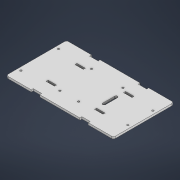
# Autodesk Inventor part: chassis
Saved by Autodesk Inventor 2021 (Build 250183000, 183)
## iProperties
Created: 2022-06-26
Part Number: chassis
Material: Generic
Document SubType Name: Modeling
Designer: phand
Density: 1 g/cm^3
Appearance: Default
Author: phand
Autodesk Inventor part; units mm, degrees
ref_plane "YZ Plane" through (0, 0, 0) normal (1, 0, 0) x (0, 1, 0)
ref_plane "XZ Plane" through (0, 0, 0) normal (0, 1, 0) x (-1, 0, 0)
ref_plane "XY Plane" through (0, 0, 0) normal (0, 0, 1) x (1, 0, 0)
sketch "Sketch1" plane through (0, 0, 0) normal (0, 1, 0) x (-1, 0, 0)
  line L0 (80, 45) -> (-80, 45)
  line L1 (-80, 45) -> (-80, -45)
  line L2 (-80, -45) -> (80, -45)
  line L3 (80, -45) -> (80, 45)
  line L4 (80, 45) -> (-80, -45) construction
  line L5 (-80, 45) -> (80, -45) construction
  point P0 (0, 0)
  dimension "d0" = 160
  dimension "d1" = 90
  constraints: 12 end point, 2 midpoint, 2 parallel, 1 horizontal, 1 perpendicular
  measures "d0" distance of L2.end L1.end
  measures "d1" distance of L1.end L0.end
extrude "Extrusion1" add sketch "Sketch1" along normal blind 3
sketch "Sketch2" plane through (0, 3, 0) normal (0, 1, 0) x (1, 0, 0)
  line L0 (-42.5, -45) -> (-30, -45)
  line L1 (-30, -45) -> (-30, -41.995)
  line L2 (-30, -41.995) -> (-42.5, -41.995)
  line L3 (-42.5, -41.995) -> (-42.5, -45)
  line L4 (-80, -45) -> (80, -45) construction
  line L5 (0, -45) -> (0, 45) construction
  line L6 (80, 45) -> (-80, 45) construction
  line L7 (-80, 45) -> (-80, -45) construction
  line L8 (-80, 0) -> (80, 0) construction
  line L9 (80, -45) -> (80, 45) construction
  line L10 (-30, -23.095) -> (-42.5, -23.095)
  line L11 (-42.5, -23.095) -> (-42.5, -20.095)
  line L12 (-42.5, -20.095) -> (-30, -20.095)
  line L13 (-30, -20.095) -> (-30, -23.095)
  line L14 (-42.5, 45) -> (-30, 45)
  line L15 (-30, 45) -> (-30, 41.995)
  line L16 (-30, 41.995) -> (-42.5, 41.995)
  line L17 (-42.5, 41.995) -> (-42.5, 45)
  line L18 (-30, 23.095) -> (-42.5, 23.095)
  line L19 (-42.5, 23.095) -> (-42.5, 20.095)
  line L20 (-42.5, 20.095) -> (-30, 20.095)
  line L21 (-30, 20.095) -> (-30, 23.095)
  line L22 (42.5, -45) -> (30, -45)
  line L23 (30, -45) -> (30, -41.995)
  line L24 (30, -41.995) -> (42.5, -41.995)
  line L25 (42.5, -41.995) -> (42.5, -45)
  line L26 (30, -23.095) -> (42.5, -23.095)
  line L27 (42.5, -23.095) -> (42.5, -20.095)
  line L28 (42.5, -20.095) -> (30, -20.095)
  line L29 (30, -20.095) -> (30, -23.095)
  line L30 (30, 45) -> (30, 41.995)
  line L31 (30, 20.095) -> (30, 23.095)
  line L32 (42.5, 45) -> (30, 45)
  line L33 (42.5, 41.995) -> (42.5, 45)
  line L34 (30, 23.095) -> (42.5, 23.095)
  line L35 (42.5, 23.095) -> (42.5, 20.095)
  line L36 (42.5, 20.095) -> (30, 20.095)
  line L37 (30, 41.995) -> (42.5, 41.995)
  point P0 (0, 0)
  point P1 (-36.25, -45)
  point P2 (-36.25, 45)
  point P3 (36.25, -45)
  point P4 (36.25, 45)
  dimension "d4" = 12.5
  dimension "d5" = 3.005
  dimension "d6" = 50
  dimension "d9" = 12.5
  dimension "d10" = 3
  dimension "d11" = 18.9
  constraints: 68 end point, 27 symmetric about line, 5 midpoint, 4 parallel, 2 horizontal, 2 perpendicular, 1 point on line
  measures "d4" distance of L2.end L1.end
  measures "d5" distance of L1.end L0.end
  measures "d6" distance between parallel lines of L7 L1
  measures "d9" distance of L11.end L12.end
  measures "d10" distance of L10.end L11.end
  measures "d11" distance between parallel lines of L10 L2
extrude "Extrusion2" cut sketch "Sketch2" against normal through all
fillet "Fillet1" radius 3 4 edges at (-80, 1.5, 45) (-80, 1.5, -45) (80, 1.5, -45) (80, 1.5, 45)
sketch "Sketch4" plane through (0, 3, 0) normal (0, 1, 0) x (1, 0, 0)
  line L0 (30, 9) -> (30, -9) construction
  line L1 (28, 9) -> (28, -9)
  line L2 (32, -9) -> (32, 9)
  arc A0 (32, 9) -> (28, 9) centre (30, 9) ccw
  arc A1 (28, -9) -> (32, -9) centre (30, -9) ccw
  line L3 (80, -42) -> (80, 42) projected
  line L4 (42.5, -45) -> (77, -45) projected
  point P0 (0, 0)
  point P1 (30, 0)
  dimension "d18" = 9
  dimension "d19" = 4
  dimension "d20" = 48
  constraints: 8 end point, 4 point on circle, 4 tangent, 2 centre point, 1 midpoint, 1 parallel, 1 vertical
  measures "d18" distance of point (30, 0) L0.end
  measures "d19" diameter of A1
  measures "d20" distance between parallel lines of L3 L2
extrude "Extrusion4" cut sketch "Sketch4" against normal through all
sketch "Sketch5" plane through (0, 3, 0) normal (0, 1, 0) x (1, 0, 0)
  circle A0 centre (75, -18.69) radius 1.4
  line L0 (80, -42) -> (80, 42) construction
  line L1 (80, 0) -> (-80, 0) construction
  line L2 (-80, 42) -> (-80, -42) construction
  circle A1 centre (75, 18.69) radius 1.4
  circle A2 centre (-75, 28) radius 1.4
  circle A3 centre (-75, -28) radius 1.4
  circle A4 centre (-19.94, -25) radius 1.4
  circle A5 centre (8, -25) radius 1.4
  line L3 (-30, -45) -> (30, -45) construction
  line L4 (8, -25) -> (23.2, -25) construction
  line L5 (23.2, -25) -> (23.2, 25.8) construction
  circle A6 centre (23.2, 25.8) radius 1.4
  line L6 (-19.94, -25) -> (-24.64, -25) construction
  line L7 (-24.64, -25) -> (-24.64, 26.9) construction
  circle A7 centre (-24.64, 26.9) radius 1.4
  line L8 (-19.94, -25) -> (8, -25) construction
  point P0 (0, 0)
  dimension "d23" = 2.8
  dimension "d24" = 18.69
  dimension "d25" = 5
  dimension "d29" = 2.8
  dimension "d30" = 5
  dimension "d31" = 28
  dimension "d32" = 2.8
  dimension "d33" = 2.8
  dimension "d40" = 15.2
  dimension "d41" = 2.8
  dimension "d43" = 4.7
  dimension "d44" = 2.8
  dimension "d46" = 27.94
  dimension "d47" = 20
  dimension "d48" = 51.9
  dimension "d49" = 50.8
  dimension "d50" = 20
  dimension "d51" = 72
  constraints: 12 end point, 8 centre point, 2 coincident, 2 horizontal, 2 midpoint, 2 symmetric about line, 2 vertical, 2 other
  measures "d23" diameter of A0
  measures "d24" distance from line of L1 A0.centre
  measures "d25" distance from line of L0 A0.centre
  measures "d29" diameter of A2
  measures "d30" distance from line of L2 A2.centre
  measures "d31" distance from line of L1 A2.centre
  measures "d32" diameter of A4
  measures "d33" diameter of A5
  measures "d40" distance of L4.start L4.end
  measures "d41" diameter of A6
  measures "d43" distance of L6.start L6.end
  measures "d44" diameter of A7
  measures "d46" distance of L4.start L6.start
  measures "d47" distance from line of L3 L6.start
  measures "d48" distance of L6.end L7.end
  measures "d49" distance of L4.end L5.end
  measures "d50" distance from line of L3 L4.start
  measures "d51" distance from line of L0 L4.start
extrude "Extrusion5" cut sketch "Sketch5" against normal through all
body "Solid1"
